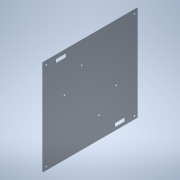
# Autodesk Inventor part: lc_box_side
Saved by Autodesk Inventor 2021.3 (Build 253353000, 353)
## iProperties
Created: 2019-07-19
Part Number: lc_box_side
Material: ポリカーボネート、クリア
Document SubType Name: Modeling
Designer: gisen
Density: 1.2 g/cm^3
Appearance: ポリカーボネート - クリア
Mass: 185.38 g
Surface Area: 1454.08 cm^2
Volume: 185.38 cm^3
Author: gisen
Autodesk Inventor part; units mm, degrees
ref_plane "YZ Plane" through (0, 0, 0) normal (1, 0, 0) x (0, 1, 0)
sketch "スケッチ1" plane through (0, 0, 0) normal (1, 0, 0) x (0, 1, 0)
  line L0 (125.6523, 179.1954) -> (-164.3477, 179.1954)
  line L1 (-164.3477, 179.1954) -> (-164.3477, -110.8046)
  line L2 (-164.3477, -110.8046) -> (125.6523, -110.8046)
  line L3 (125.6523, -110.8046) -> (125.6523, 179.1954)
  point P0 (0, 0)
  dimension "d0" = 290
  dimension "d1" = 290
  constraints: 8 end point, 2 parallel, 1 horizontal, 1 perpendicular
  measures "d0" distance of L0.start L0.end
  measures "d1" distance of L2.end L0.start
extrude "押し出し1" add sketch "スケッチ1" along normal blind 2.6
sketch "スケッチ2" plane through (2.6, 0, 0) normal (1, 0, 0) x (0, 0, -1)
  line L0 (-179.1954, 125.6523) -> (-179.1954, -164.3477) projected
  line L1 (-179.1954, -164.3477) -> (110.8046, -164.3477) projected
  line L2 (110.8046, -164.3477) -> (110.8046, 125.6523) projected
  line L3 (110.8046, 125.6523) -> (-179.1954, 125.6523) projected
  line L4 (-34.1954, -19.3477) -> (-34.1954, 125.6523)
  line L5 (110.8046, 125.6523) -> (-179.1954, 125.6523) projected
  line L6 (-34.1954, -19.3477) -> (110.8046, -19.3477)
  point P0 (0, 0)
  point P1 (-169.1954, 115.6523)
  point P2 (100.8046, 115.6523)
  point P3 (-169.1954, -154.3477)
  point P4 (100.8046, -154.3477)
  dimension "d4" = 10
  dimension "d5" = 10
  constraints: 4 end point, 3 symmetric about line, 2 midpoint
  measures "d4" distance from line of L3 point (-169.195, 115.652)
  measures "d5" distance from line of L0 point (-169.195, 115.652)
hole "穴1" at (2.6, 115.6523, 169.1954) at (2.6, 115.6523, -100.8046) at (2.6, -154.3477, 169.1954) at (2.6, -154.3477, -100.8046) direction (-1, 0, 0) diameter 4.5 depth 10 tip angle 118
sketch "スケッチ4" plane through (0, 0, 0) normal (-1, 0, 0) x (0, 0, 1)
  line L0 (179.1954, -164.3477) -> (-110.8046, -164.3477) projected
  line L1 (-110.8046, -164.3477) -> (-110.8046, 125.6523) projected
  line L2 (-110.8046, 126.1523) -> (179.1954, 126.1523) projected
  circle A0 centre (169.1954, -154.3477) radius 2.25 projected
  circle A1 centre (169.1954, 115.6523) radius 2.25 projected
  circle A2 centre (-100.8046, 115.6523) radius 2.25 projected
  circle A3 centre (-100.8046, -154.3477) radius 2.25 projected
  line L3 (179.1954, 125.6523) -> (179.1954, -164.3477) projected
  line L4 (-110.8046, 125.6523) -> (179.1954, 125.6523) projected
  line L5 (-110.8046, -164.3477) -> (-110.8046, 125.6523) projected
  line L6 (179.1954, -164.3477) -> (-110.8046, -164.3477) projected
  line L7 (179.1954, -164.3477) -> (-110.8046, -164.3477) projected
  line L8 (-70.8046, -152.3477) -> (-70.8046, -146.3477)
  line L9 (-68.8046, -144.3477) -> (-42.8046, -144.3477)
  line L10 (-40.8046, -146.3477) -> (-40.8046, -152.3477)
  arc A4 (-68.8046, -144.3477) -> (-70.8046, -146.3477) centre (-68.8046, -146.3477) ccw
  arc A5 (-40.8046, -146.3477) -> (-42.8046, -144.3477) centre (-42.8046, -146.3477) ccw
  line L11 (-42.8046, -154.3477) -> (-68.8046, -154.3477)
  arc A6 (-42.8046, -154.3477) -> (-40.8046, -152.3477) centre (-42.8046, -152.3477) ccw
  arc A7 (-70.8046, -152.3477) -> (-68.8046, -154.3477) centre (-68.8046, -152.3477) ccw
  arc A8 (109.1954, 107.6523) -> (111.1954, 105.6523) centre (111.1954, 107.6523) ccw
  line L12 (109.1954, 107.6523) -> (109.1954, 113.6523)
  arc A9 (111.1954, 115.6523) -> (109.1954, 113.6523) centre (111.1954, 113.6523) ccw
  line L13 (111.1954, 115.6523) -> (137.1954, 115.6523)
  line L14 (137.1954, 105.6523) -> (111.1954, 105.6523)
  arc A10 (137.1954, 105.6523) -> (139.1954, 107.6523) centre (137.1954, 107.6523) ccw
  line L15 (139.1954, 113.6523) -> (139.1954, 107.6523)
  arc A11 (139.1954, 113.6523) -> (137.1954, 115.6523) centre (137.1954, 113.6523) ccw
  point P0 (0, 0)
  point P1 (-70.8046, -164.3477)
  point P2 (-70.8046, -144.3477)
  point P3 (-40.8046, -144.3477)
  point P4 (-40.8046, -164.3477)
  point P5 (34.1954, -19.3477)
  point P6 (109.1954, 105.6523)
  point P7 (109.1954, 125.6523)
  point P8 (139.1954, 105.6523)
  point P9 (139.1954, 125.6523)
  dimension "d19" = 40
  dimension "d20" = 30
  dimension "d21" = 20
  dimension "d22" = 2
  dimension "d23" = 10
  dimension "d24" = 2
  dimension "d25" = 145
  dimension "d26" = 145
  dimension "d29" = 360
  constraints: 16 end point, 16 point on circle, 14 point on line, 8 centre point, 8 tangent, 4 perpendicular, 2 equal radius, 49 other
  measures "d19" distance between parallel lines of L8 L1
  measures "d20" distance of point (-70.805, -144.348) point (-40.805, -144.348)
  measures "d21" distance of point (-70.805, -164.348) point (-70.805, -144.348)
  measures "d22" radius of A4
  measures "d23" distance between parallel lines of L0 L11
  measures "d24" radius of A6
  measures "d25" distance from line of L0 point (34.195, -19.348)
  measures "d26" distance from line of L3 point (34.195, -19.348)
extrude "押し出し3" cut sketch "スケッチ4" against normal blind 2.6 contours L8 A4 L9 A5 L10 A6 L11 A7 | L12 A9 L13 A11 L15 A10 L14 A8
ref_plane "作業平面4" through (2.6, 125.6523, 179.1954) normal (0, -0.7071, 0.7071) x (-1, 0, 0)
ref_plane "作業平面5" through (0, -164.3477, 179.1954) normal (0, -0.7071, -0.7071) x (0, 0.7071, -0.7071)
sketch "スケッチ5" plane through (0, 0, 0) normal (-1, 0, 0) x (0, 0, 1)
  circle A0 centre (60.7119, 60.2018) radius 1.65 projected
  circle A1 centre (113.7449, 7.1688) radius 1.65 projected
  circle A2 centre (-45.3541, -45.8642) radius 1.65 projected
  circle A3 centre (7.6789, -98.8972) radius 1.65 projected
  circle A4 centre (7.6789, -98.8972) radius 1.65 projected
  circle A5 centre (7.6789, -98.8972) radius 1.65 projected
  point P0 (0, 0)
  constraints: 4 coincident
hole "穴2" at (0, 7.1688, 113.7449) at (0, -98.8972, 7.6789) at (0, -45.8642, -45.3541) at (0, 60.2018, 60.7119) at (0, 7.1688, 113.7449) direction (1, 0, 0) diameter 4.5 end through all
